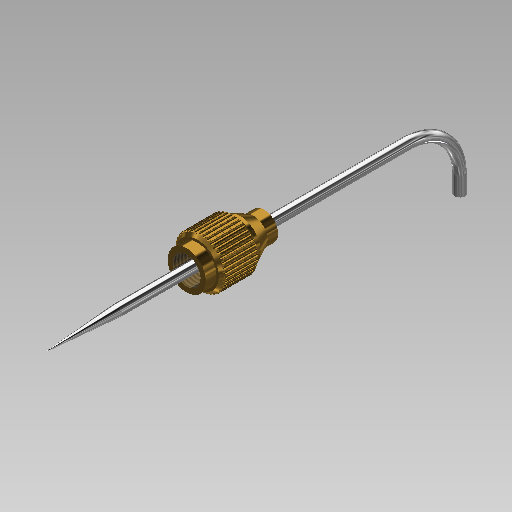
# Autodesk Inventor part: throttle
Saved by Autodesk Inventor 2018.1 (Build 221171000, 171)
## iProperties
Created: 2013-08-26
Part Number: throttle
Material: Generic
Document SubType Name: Modeling
Designer: Konstantin
Density: 1 g/cm^3
Appearance: Default
Mass: 0.338179 g
Surface Area: 6.58043 cm^2
Volume: 0.338179 cm^3
Author: Konstantin
Autodesk Inventor part; units mm, degrees
ref_plane "YZ Plane" through (0, 0, 0) normal (1, 0, 0) x (0, 1, 0)
ref_plane "XZ Plane" through (0, 0, 0) normal (0, 1, 0) x (-1, 0, 0)
ref_plane "XY Plane" through (0, 0, 0) normal (0, 0, 1) x (1, 0, 0)
sketch "Sketch2" plane through (0, 0, 0) normal (0, 0, 1) x (1, 0, 0)
  arc A0 (-0.2228, 3.6432) -> (0.2228, 3.6432) centre (0, 3.6432) ccw
  arc A1 (-0.79, 3.5635) -> (-0.3498, 3.6332) centre (-0.5699, 3.5983) ccw
  arc A2 (-1.3377, 3.396) -> (-0.9139, 3.5337) centre (-1.1258, 3.4649) ccw
  arc A3 (-1.8525, 3.1449) -> (-1.4554, 3.3473) centre (-1.654, 3.2461) ccw
  arc A4 (-2.3217, 2.8164) -> (-1.9611, 3.0784) centre (-2.1414, 2.9474) ccw
  arc A5 (-2.7337, 2.4186) -> (-2.4186, 2.7337) centre (-2.5761, 2.5761) ccw
  arc A6 (-3.0784, 1.9611) -> (-2.8164, 2.3217) centre (-2.9474, 2.1414) ccw
  arc A7 (-3.3473, 1.4554) -> (-3.1449, 1.8525) centre (-3.2461, 1.654) ccw
  arc A8 (-3.5337, 0.9139) -> (-3.396, 1.3377) centre (-3.4649, 1.1258) ccw
  arc A9 (-3.6332, 0.3498) -> (-3.5635, 0.79) centre (-3.5983, 0.5699) ccw
  arc A10 (-3.6432, -0.2228) -> (-3.6432, 0.2228) centre (-3.6432, 0) ccw
  arc A11 (-3.5635, -0.79) -> (-3.6332, -0.3498) centre (-3.5983, -0.5699) ccw
  arc A12 (-3.396, -1.3377) -> (-3.5337, -0.9139) centre (-3.4649, -1.1258) ccw
  arc A13 (-3.1449, -1.8525) -> (-3.3473, -1.4554) centre (-3.2461, -1.654) ccw
  arc A14 (-2.8164, -2.3217) -> (-3.0784, -1.9611) centre (-2.9474, -2.1414) ccw
  arc A15 (-2.4186, -2.7337) -> (-2.7337, -2.4186) centre (-2.5761, -2.5761) ccw
  arc A16 (-1.9611, -3.0784) -> (-2.3217, -2.8164) centre (-2.1414, -2.9474) ccw
  arc A17 (-1.4554, -3.3473) -> (-1.8525, -3.1449) centre (-1.654, -3.2461) ccw
  arc A18 (-0.9139, -3.5337) -> (-1.3377, -3.396) centre (-1.1258, -3.4649) ccw
  arc A19 (-0.3498, -3.6332) -> (-0.79, -3.5635) centre (-0.5699, -3.5983) ccw
  arc A20 (0.2228, -3.6432) -> (-0.2228, -3.6432) centre (0, -3.6432) ccw
  arc A21 (0.79, -3.5635) -> (0.3498, -3.6332) centre (0.5699, -3.5983) ccw
  arc A22 (1.3377, -3.396) -> (0.9139, -3.5337) centre (1.1258, -3.4649) ccw
  arc A23 (1.8525, -3.1449) -> (1.4554, -3.3473) centre (1.654, -3.2461) ccw
  arc A24 (2.3217, -2.8164) -> (1.9611, -3.0784) centre (2.1414, -2.9474) ccw
  arc A25 (2.7337, -2.4186) -> (2.4186, -2.7337) centre (2.5761, -2.5761) ccw
  arc A26 (3.0784, -1.9611) -> (2.8164, -2.3217) centre (2.9474, -2.1414) ccw
  arc A27 (3.3473, -1.4554) -> (3.1449, -1.8525) centre (3.2461, -1.654) ccw
  arc A28 (3.5337, -0.9139) -> (3.396, -1.3377) centre (3.4649, -1.1258) ccw
  arc A29 (3.6332, -0.3498) -> (3.5635, -0.79) centre (3.5983, -0.5699) ccw
  arc A30 (3.6432, 0.2228) -> (3.6432, -0.2228) centre (3.6432, 0) ccw
  arc A31 (3.5635, 0.79) -> (3.6332, 0.3498) centre (3.5983, 0.5699) ccw
  arc A32 (3.396, 1.3377) -> (3.5337, 0.9139) centre (3.4649, 1.1258) ccw
  arc A33 (3.1449, 1.8525) -> (3.3473, 1.4554) centre (3.2461, 1.654) ccw
  arc A34 (2.8164, 2.3217) -> (3.0784, 1.9611) centre (2.9474, 2.1414) ccw
  arc A35 (2.4186, 2.7337) -> (2.7337, 2.4186) centre (2.5761, 2.5761) ccw
  arc A36 (1.9611, 3.0784) -> (2.3217, 2.8164) centre (2.1414, 2.9474) ccw
  arc A37 (1.4554, 3.3473) -> (1.8525, 3.1449) centre (1.654, 3.2461) ccw
  arc A38 (0.9139, 3.5337) -> (1.3377, 3.396) centre (1.1258, 3.4649) ccw
  arc A39 (0.3498, 3.6332) -> (0.79, 3.5635) centre (0.5699, 3.5983) ccw
  arc A40 (-0.2228, 3.6432) -> (-0.3498, 3.6332) centre (0, 0) ccw
  arc A41 (-0.79, 3.5635) -> (-0.9139, 3.5337) centre (0, 0) ccw
  arc A42 (0.3498, 3.6332) -> (0.2228, 3.6432) centre (0, 0) ccw
  arc A43 (0.9139, 3.5337) -> (0.79, 3.5635) centre (0, 0) ccw
  arc A44 (1.4554, 3.3473) -> (1.3377, 3.396) centre (0, 0) ccw
  arc A45 (-1.3377, 3.396) -> (-1.4554, 3.3473) centre (0, 0) ccw
  arc A46 (-1.8525, 3.1449) -> (-1.9611, 3.0784) centre (0, 0) ccw
  arc A47 (-2.3217, 2.8164) -> (-2.4186, 2.7337) centre (0, 0) ccw
  arc A48 (-2.7337, 2.4186) -> (-2.8164, 2.3217) centre (0, 0) ccw
  arc A49 (-3.0784, 1.9611) -> (-3.1449, 1.8525) centre (0, 0) ccw
  arc A50 (-3.3473, 1.4554) -> (-3.396, 1.3377) centre (0, 0) ccw
  arc A51 (-3.5337, 0.9139) -> (-3.5635, 0.79) centre (0, 0) ccw
  arc A52 (-3.6332, 0.3498) -> (-3.6432, 0.2228) centre (0, 0) ccw
  arc A53 (-3.6432, -0.2228) -> (-3.6332, -0.3498) centre (0, 0) ccw
  arc A54 (-3.5635, -0.79) -> (-3.5337, -0.9139) centre (0, 0) ccw
  arc A55 (-3.396, -1.3377) -> (-3.3473, -1.4554) centre (0, 0) ccw
  arc A56 (-3.1449, -1.8525) -> (-3.0784, -1.9611) centre (0, 0) ccw
  arc A57 (-2.8164, -2.3217) -> (-2.7337, -2.4186) centre (0, 0) ccw
  arc A58 (1.9611, 3.0784) -> (1.8525, 3.1449) centre (0, 0) ccw
  arc A59 (2.4186, 2.7337) -> (2.3217, 2.8164) centre (0, 0) ccw
  arc A60 (2.8164, 2.3217) -> (2.7337, 2.4186) centre (0, 0) ccw
  arc A61 (3.1449, 1.8525) -> (3.0784, 1.9611) centre (0, 0) ccw
  arc A62 (3.396, 1.3377) -> (3.3473, 1.4554) centre (0, 0) ccw
  arc A63 (3.5635, 0.79) -> (3.5337, 0.9139) centre (0, 0) ccw
  arc A64 (3.6432, 0.2228) -> (3.6332, 0.3498) centre (0, 0) ccw
  arc A65 (3.6332, -0.3498) -> (3.6432, -0.2228) centre (0, 0) ccw
  arc A66 (3.5337, -0.9139) -> (3.5635, -0.79) centre (0, 0) ccw
  arc A67 (3.3473, -1.4554) -> (3.396, -1.3377) centre (0, 0) ccw
  arc A68 (3.0784, -1.9611) -> (3.1449, -1.8525) centre (0, 0) ccw
  arc A69 (2.7337, -2.4186) -> (2.8164, -2.3217) centre (0, 0) ccw
  arc A70 (2.3217, -2.8164) -> (2.4186, -2.7337) centre (0, 0) ccw
  arc A71 (1.8525, -3.1449) -> (1.9611, -3.0784) centre (0, 0) ccw
  arc A72 (1.3377, -3.396) -> (1.4554, -3.3473) centre (0, 0) ccw
  arc A73 (0.79, -3.5635) -> (0.9139, -3.5337) centre (0, 0) ccw
  arc A74 (0.2228, -3.6432) -> (0.3498, -3.6332) centre (0, 0) ccw
  arc A75 (-0.3498, -3.6332) -> (-0.2228, -3.6432) centre (0, 0) ccw
  arc A76 (-0.9139, -3.5337) -> (-0.79, -3.5635) centre (0, 0) ccw
  arc A77 (-1.4554, -3.3473) -> (-1.3377, -3.396) centre (0, 0) ccw
  arc A78 (-2.4186, -2.7337) -> (-2.3217, -2.8164) centre (0, 0) ccw
  arc A79 (-1.9611, -3.0784) -> (-1.8525, -3.1449) centre (0, 0) ccw
  dimension "d16" = 360
  constraints: 80 point on circle, 40 centre point, 283 other
extrude "Extrusion1" add sketch "Sketch2" along normal blind 5.6
sketch "Sketch3" plane through (0, 0, 5.6) normal (0, 0, 1) x (1, 0, 0)
  circle A0 centre (0, 0) radius 2.75
  constraints: 1 centre point, 1 other
extrude "Extrusion2" add sketch "Sketch3" along normal blind 1.5
sketch "Sketch4" plane through (0, 0, 0) normal (1, 0, 0) x (0, 1, 0)
  line L0 (3.8682, 5.825) -> (3.8682, 4.825)
  line L1 (3.8682, 0.775) -> (3.8682, -0.225)
  line L2 (3.8682, 5.825) -> (2.8682, 5.825)
  line L3 (3.8682, -0.225) -> (2.8682, -0.225)
  line L4 (2.8682, 5.825) -> (3.8682, 4.825)
  line L5 (2.8682, -0.225) -> (3.8682, 0.775)
  line L6 (0, 7.1) -> (0, 8.2561) construction
  dimension "d26" = 2.4311
  dimension "d27" = 1.275
  constraints: 14 end point, 3 vertical, 2 horizontal, 2 perpendicular, 1 parallel, 2 other
  measures "d26" distance from line of L6.end L2
  measures "d27" distance from line of L6.start L2
revolve "Revolution1" cut sketch "Sketch4" angle 360 about axis through (0, 0, 7.1) along (0, 0, 1)
sketch "Sketch5" plane through (0, 0, 0) normal (0, 0, -1) x (-1, 0, 0)
  circle A0 centre (0, 0) radius 3
  dimension "d29" = 6
  constraints: 1 centre point, 1 coincident
  measures "d29" diameter of A0
extrude "Extrusion3" add sketch "Sketch5" along normal blind 2.5
chamfer "Chamfer1" distance 1 distance2 2 1 edges at (3, 0, -2.5) measured on face at (0.7485, 1.2069, -2.5)
sketch "Sketch6" plane through (0, 0, -2.5) normal (0, 0, -1) x (-1, 0, 0)
  circle A0 centre (0, 0) radius 2 projected
extrude "Extrusion4" add sketch "Sketch6" along normal blind 1.5
sketch "Sketch7" plane through (0, 0, 7.1) normal (0, 0, 1) x (1, 0, 0)
  circle A0 centre (0, 0) radius 0.5
  dimension "d37" = 1
  constraints: 1 centre point, 1 coincident
  measures "d37" diameter of A0
hole "Hole1" at (0, 0, 7.1) direction (0, 0, -1) diameter 4 depth 6 tip angle 118
thread "Thread1"
sketch "Sketch9" plane through (0, 0, 7.1) normal (0, 0, 1) x (1, 0, 0)
  circle A0 centre (0, 0) radius 0.75
  constraints: 1 centre point, 1 other
sketch3d "3D Sketch1"
  line L0 (0, 0, 27.1) -> (0, 0, -24.5012)
  arc A0 (0, 0, -24.5012) -> (0, -7.5, -32.0012) centre (0, -7.5, -24.5012) ccw
  line L1 (0, -7.5, -32.0012) -> (0, -9.9981, -32.0012)
  dimension "d55" = 7.5
sweep "Sweep1" add profiles "Sketch9" path "3D Sketch1"
chamfer "Chamfer2" distance 10 distance2 0.7 1 edges at (-0.75, 0, 27.1) measured on face at (-0.092, -0.7443, 9.2659)
body "Solid1"
